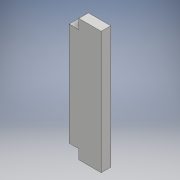
# Autodesk Inventor part: muñeca2
Saved by Autodesk Inventor 2018 (Build 220112000, 112)
## iProperties
Created: 2020-03-11
Part Number: muñeca2
Material: Genérico
Document SubType Name: Modeling
Designer: david
Density: 1 g/cm^3
Appearance: Valor por defecto
Author: david
Autodesk Inventor part; units mm, degrees
ref_plane "YZ Plane" through (0, 0, 0) normal (1, 0, 0) x (0, 1, 0)
ref_plane "XZ Plane" through (0, 0, 0) normal (0, 1, 0) x (-1, 0, 0)
ref_plane "XY Plane" through (0, 0, 0) normal (0, 0, 1) x (1, 0, 0)
sketch "Boceto1" plane through (0, 0, 0) normal (0, 1, 0) x (-1, 0, 0)
  line L0 (10, 0) -> (10, -26.35)
  line L1 (0, -26.35) -> (0, 0)
  line L2 (0, 0) -> (0, 3)
  line L3 (0, 3) -> (10, 3)
  line L4 (10, 3) -> (10, 0)
  line L5 (10, -26.35) -> (10, -29.35)
  line L6 (10, -29.35) -> (0, -29.35)
  line L7 (0, -29.35) -> (0, -26.35)
  constraints: 16 end point, 3 perpendicular, 2 vertical, 1 collinear
extrude "Extrusión1" add sketch "Boceto1" along normal blind 3
sketch "Boceto3" plane through (0, 0, 0) normal (0, -1, 0) x (1, 0, 0)
  line L0 (0, 3) -> (0, 6)
  line L1 (0, 6) -> (-7, 6)
  line L2 (-7, 6) -> (-7, 3)
  line L3 (-7, 3) -> (0, 3)
  line L4 (0, -29.35) -> (0, -32.35)
  line L5 (0, -32.35) -> (-7, -32.35)
  line L6 (-7, -32.35) -> (-7, -29.35)
  line L7 (0, -29.35) -> (-7, -29.35)
  point P0 (0, 0)
  constraints: 16 end point, 5 perpendicular, 2 vertical
extrude "Extrusión3" add sketch "Boceto3" against normal blind 3
